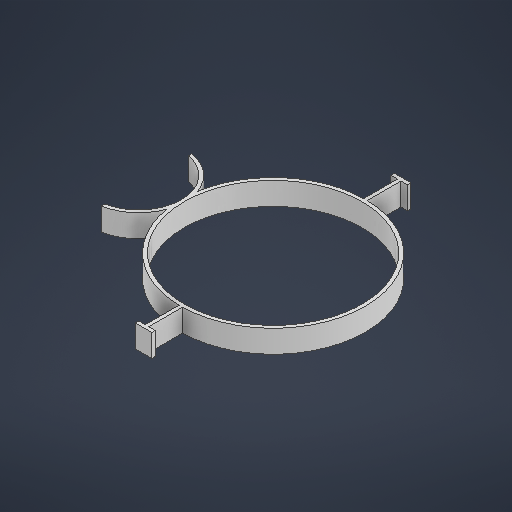
# Autodesk Inventor part: Hardware_container_foot
Saved by Autodesk Inventor 2026.1 (Build 301233000, 233)
## iProperties
Created: 2025-07-22
Part Number: Hardware_container_foot
Material: Generic
Document SubType Name: Modeling
Designer: nuiro
Density: 1 g/cm^3
Appearance: Default
Author: nuiro
Autodesk Inventor part; units mm, degrees
ref_plane "YZ Plane" through (0, 0, 0) normal (1, 0, 0) x (0, 1, 0)
ref_plane "XZ Plane" through (0, 0, 0) normal (0, 1, 0) x (-1, 0, 0)
ref_plane "XY Plane" through (0, 0, 0) normal (0, 0, 1) x (1, 0, 0)
sketch "Sketch1" plane through (0, 0, 0) normal (0, 1, 0) x (-1, 0, 0)
  circle A0 centre (0, 0) radius 51.25
  arc A1 (73, 24.0832) -> (73, -24.0832) centre (77.5, 0) ccw
  line L0 (73, -26.1151) -> (73, -24.0832)
  line L1 (73, 24.0832) -> (73, 26.1151)
  line L2 (1, 74.75) -> (-1, 74.75)
  line L3 (-1, -74.75) -> (1, -74.75)
  line L4 (4.75, 74.7472) -> (-4.75, 74.7472)
  line L5 (-4.75, 74.7472) -> (-4.75, 72.7472)
  line L6 (4.75, 72.7472) -> (4.75, 74.7472)
  line L7 (4.75, -74.75) -> (-4.75, -74.75)
  line L8 (-4.75, -74.75) -> (-4.75, -72.75)
  line L9 (4.75, -72.75) -> (4.75, -74.75)
  line L10 (1, -72.75) -> (1, -53.2406)
  line L11 (-1, -53.2406) -> (-1, -72.75)
  line L12 (-1, 74.75) -> (-1, 74.7472)
  line L13 (-1, 72.7472) -> (-1, 53.2406)
  line L14 (1, 53.2406) -> (1, 72.7472)
  line L15 (1, 74.7472) -> (1, 74.75)
  line L16 (-4.75, 72.7472) -> (-1, 72.7472)
  line L17 (1, 72.7472) -> (4.75, 72.7472)
  line L18 (-4.75, -72.75) -> (-1, -72.75)
  line L19 (1, -72.75) -> (4.75, -72.75)
  arc A2 (73, 26.1151) -> (52.5133, 8.827) centre (77.5, 0) ccw
  arc A3 (52.5133, -8.827) -> (73, -26.1151) centre (77.5, 0) ccw
  arc A4 (1, -53.2406) -> (52.5133, -8.827) centre (0, 0) ccw
  arc A5 (52.5133, 8.827) -> (1, 53.2406) centre (0, 0) ccw
  arc A6 (-1, 53.2406) -> (-1, -53.2406) centre (0, 0) ccw
  point P0 (-4.75, 73.7472)
  dimension "d0" = 102.5
  dimension "d2" = 77.5
  dimension "d3" = 49
  dimension "d11" = 149.5
  dimension "d12" = 74.75
  dimension "d13" = 9.5
  dimension "d18" = 9.5
  constraints: 40 end point, 16 parallel, 12 point on circle, 7 centre point, 5 perpendicular, 3 coincident, 3 horizontal, 2 point on line, 1 midpoint
  measures "d0" diameter of A0
  measures "d2" distance of point (0, 0) A1.centre
  measures "d3" diameter of A1
  measures "d11" distance between parallel lines of L2 L3
  measures "d12" distance from line of point (0, 0) L2
  measures "d13" distance between parallel lines of L5 L6
  measures "d18" distance between parallel lines of L8 L9
extrude "Extrusion1" add sketch "Sketch1" along normal blind 13 contours A1 L0 A3 A4 L10 L19 L9 L7 L3 L8 L18 L11 A6 L13 L16 L5 L4 L6 L17 L14 A5 A2 L1
body "Solid1"
